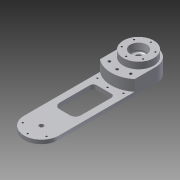
# Autodesk Inventor part: JointC2_2nd
Saved by Autodesk Inventor 2013 (Build 170138000, 138)
## iProperties
Created: 2013-02-07
Part Number: JointC2_2nd
Document SubType Name: Modeling
Designer: JohnHenry
Density: 0.899 g/cm^3
Material: ポリプロピレン
Mass: 21.971 g
Surface Area: 103.887 cm^2
Volume: 24.4394 cm^3
Author: JohnHenry
Autodesk Inventor part; units mm, degrees
ref_plane "YZ Plane" through (0, 0, 0) normal (1, 0, 0) x (0, 1, 0)
ref_plane "XZ Plane" through (0, 0, 0) normal (0, 1, 0) x (-1, 0, 0)
ref_plane "XY Plane" through (0, 0, 0) normal (0, 0, 1) x (1, 0, 0)
sketch "スケッチ1" plane through (0, 0, 0) normal (0, 0, 1) x (1, 0, 0)
  line L0 (-15.75, -60) -> (15.75, -60)
  line L1 (15.75, -60) -> (15.75, 60)
  line L2 (15.75, 60) -> (-15.75, 60)
  line L3 (-15.75, 60) -> (-15.75, -60)
  point P0 (0, 0)
  dimension "d0" = 31.5
  dimension "d1" = 15.75
  dimension "d2" = 120
  dimension "d3" = 60
  constraints: 8 end point, 2 parallel, 1 horizontal, 1 perpendicular
  measures "d0" distance of L1.end L2.end
  measures "d1" distance from line of L1 point (0, 0)
  measures "d2" distance of L2.end L0.start
  measures "d3" distance from line of L0 point (0, 0)
extrude "押し出し1" add sketch "スケッチ1" along normal blind 5
fillet "フィレット1" radius 15.75 4 edges at (-15.75, 60, 2.5) (15.75, 60, 2.5) (15.75, -60, 2.5) (-15.75, -60, 2.5)
sketch "スケッチ2" plane through (0, 0, 5) normal (0, 0, 1) x (1, 0, 0)
  arc A0 (15.75, 44.25) -> (-15.75, 44.25) centre (0, 44.25) ccw projected
  circle A1 centre (0, 44.25) radius 11.25
  point P0 (0, 0)
  point P1 (0, 55.5)
  point P2 (9.7428, 49.875)
  point P3 (9.7428, 38.625)
  point P4 (0, 33)
  point P5 (-9.7428, 38.625)
  point P6 (-9.7428, 49.875)
  dimension "d7" = 22.5
  dimension "d10" = 360
  constraints: 1 coincident, 1 vertical alignment, 9 other
hole "Hole1" at (0, 55.5, 5) at (9.7428, 49.875, 5) at (9.7428, 38.625, 5) at (0, 33, 5) at (-9.7428, 38.625, 5) at (-9.7428, 49.875, 5) direction (0, 0, -1) diameter 1.567 depth 8 tip angle 118 thread size "M2x0.4" class "6H" standard "ISO Metric profile"
sketch "スケッチ3" plane through (0, 0, 5) normal (0, 0, 1) x (1, 0, 0)
  arc A0 (15.75, 44.25) -> (-15.75, 44.25) centre (0, 44.25) ccw projected
  point P0 (0, 0)
  constraints: 1 coincident
hole "Hole2" at (0, 44.25, 5) direction (0, 0, -1) diameter 13 end through all
chamfer "面取り1" distance 1 distance2 5 1 edges at (0, 50.75, 5) measured on face at (0, -18.7612, 5)
sketch "スケッチ5" plane through (0, 0, 0) normal (0, 0, -1) x (-1, 0, 0)
  circle A0 centre (9.7428, 49.875) radius 0.7835 projected
  circle A1 centre (9.7428, 38.625) radius 0.7835 projected
  circle A2 centre (0, 33) radius 0.7835 projected
  circle A3 centre (-9.7428, 38.625) radius 0.7835 projected
  circle A4 centre (-9.7428, 49.875) radius 0.7835 projected
  circle A5 centre (0, 55.5) radius 0.7835 projected
  arc A6 (-15.75, -44.25) -> (15.75, -44.25) centre (0, -44.25) ccw projected
  line L0 (15.75, 44.25) -> (15.75, -44.25) projected
  arc A7 (15.75, 44.25) -> (-15.75, 44.25) centre (0, 44.25) ccw projected
  line L1 (-15.75, -44.25) -> (-15.75, 44.25) projected
  circle A8 centre (0, 44.25) radius 3
  point P0 (0, 0)
  dimension "d31" = 6
  constraints: 1 centre point, 1 coincident
  measures "d31" diameter of A8
extrude "押し出し3" add sketch "スケッチ5" along normal blind 15
sketch "スケッチ6" plane through (0, 44.25, 0) normal (0, 0, 1) x (1, 0, 0)
  circle A0 centre (0, 0) radius 3 projected
  circle A1 centre (0, 0) radius 6.5 projected
  point P0 (0, -44.25)
extrude "押し出し4" cut sketch "スケッチ6" against normal blind 1
sketch "スケッチ7" plane through (0, 44.25, -1) normal (0, 0, 1) x (1, 0, 0)
  circle A0 centre (0, 0) radius 6.5 projected
  circle A1 centre (0, 0) radius 4.5
  point P0 (0, -44.25)
  dimension "d36" = 9
  constraints: 1 centre point, 1 coincident
  measures "d36" diameter of A1
extrude "押し出し5" cut sketch "スケッチ7" against normal blind 1
fillet "フィレット2" radius 1 2 edges at (-6.5, 44.25, -2) (-4.5, 44.25, -2)
sketch "スケッチ9" plane through (0, 0, 5) normal (0, 0, 1) x (1, 0, 0)
  arc A0 (-15.75, -44.25) -> (15.75, -44.25) centre (0, -44.25) ccw projected
  line L0 (15.75, 44.25) -> (15.75, -44.25) projected
  arc A1 (15.75, 44.25) -> (-15.75, 44.25) centre (0, 44.25) ccw projected
  line L1 (-15.75, -44.25) -> (-15.75, 44.25) projected
  circle A2 centre (0, 44.25) radius 7.5 projected
  circle A3 centre (0, 44.25) radius 13.9
  point P0 (0, 0)
  dimension "d46" = 27.8
  constraints: 1 centre point, 1 coincident
  measures "d46" diameter of A3
extrude "押し出し7" cut sketch "スケッチ9" against normal blind 6 contours L1 A1 L0 A0
sketch "スケッチ10" plane through (0, 0, -1) normal (0, 0, 1) x (1, 0, 0)
  line L0 (15.75, 44.25) -> (15.75, -44.25) projected
  arc A0 (15.75, 44.25) -> (-15.75, 44.25) centre (0, 44.25) ccw projected
  line L1 (-15.75, -44.25) -> (-15.75, 44.25) projected
  arc A1 (-15.75, -44.25) -> (15.75, -44.25) centre (0, -44.25) ccw projected
  arc A2 (15.75, 24.8351) -> (-15.75, 24.8351) centre (0, 44.25) ccw
  arc A3 (-15.75, 24.8351) -> (15.75, 24.8351) centre (0, 44.25) ccw
  point P0 (0, 0)
  dimension "d49" = 50
  constraints: 4 point on circle, 2 centre point, 2 point on line, 1 coincident
  measures "d49" diameter of A2
extrude "押し出し8" cut sketch "スケッチ10" against normal blind 10 contours L0 A1 L1 A3
sketch "スケッチ11" plane through (0, 0, -11) normal (0, 0, 1) x (1, 0, 0)
  arc A0 (-15.75, -44.25) -> (15.75, -44.25) centre (0, -44.25) ccw projected
  point P0 (0, 0)
  constraints: 1 coincident
hole "Hole3" at (0, -44.25, -11) direction (0, 0, -1) diameter 4 end through all
sketch "スケッチ12" plane through (0, 0, -1) normal (0, 0, 1) x (1, 0, 0)
  line L0 (-15.75, 24.8351) -> (-15.75, 44.25) projected
  circle A0 centre (0, 44.25) radius 13.9 projected
  circle A1 centre (0, 44.25) radius 19.5
  line L1 (0, 44.25) -> (0, 63.75)
  line L2 (0, 44.25) -> (-9.75, 27.3625)
  line L3 (0, 44.25) -> (9.75, 27.3625)
  line L4 (15.75, 44.25) -> (15.75, 24.8351) projected
  arc A2 (15.75, 44.25) -> (-15.75, 44.25) centre (0, 44.25) ccw projected
  line L5 (0, 44.25) -> (0, 24.75)
  point P0 (0, 0)
  dimension "d59" = 39
  dimension "d60" = 150
  dimension "d61" = 150
  constraints: 8 end point, 4 coincident, 4 point on circle, 2 parallel, 1 centre point
  measures "d59" diameter of A1
  measures "d60" angle of L2 L1
  measures "d61" angle of L3 L1
hole "Hole4" at (-9.75, 27.3625, -1) at (9.75, 27.3625, -1) at (0, 24.75, -1) direction (0, 0, -1) diameter 2.459 end through all thread size "M3x0.5" class "6H" standard "ISO Metric profile"
sketch "スケッチ14" plane through (0, 0, -11) normal (0, 0, 1) x (1, 0, 0)
  circle A0 centre (0, -44.25) radius 2 projected
  arc A1 (-15.75, 24.8351) -> (15.75, 24.8351) centre (0, 44.25) ccw projected
  arc A2 (-15.75, -44.25) -> (15.75, -44.25) centre (0, -44.25) ccw projected
  line L0 (-9.85, 12.8) -> (9.85, 12.8)
  line L1 (9.85, 12.8) -> (9.85, -23.1)
  line L2 (9.85, -23.1) -> (-9.85, -23.1)
  line L3 (-9.85, -23.1) -> (-9.85, 12.8)
  line L4 (0, 19.25) -> (0, -60)
  point P0 (0, 0)
  dimension "d77" = 19.7
  dimension "d78" = 19.7
  dimension "d79" = 35.9
  dimension "d80" = 21.15
  constraints: 10 end point, 2 parallel, 2 point on circle, 1 horizontal, 1 perpendicular
  measures "d77" distance of L0.start L0.end
  measures "d78" diameter of L1 L4
  measures "d79" distance between parallel lines of L2 L0
  measures "d80" distance from line of A0.centre L2
extrude "押し出し9" cut sketch "スケッチ14" against normal through all contours L0 L4 L2 L3 | L0 L1 L2 L4
fillet "フィレット3" radius 5.05 2 edges at (-9.85, -23.1, -13) (9.85, -23.1, -13)
fillet "フィレット4" radius 3.05 2 edges at (-9.85, 12.8, -13) (9.85, 12.8, -13)
sketch "スケッチ15" plane through (0, 0, -11) normal (0, 0, 1) x (1, 0, 0)
  line L0 (-6.8, 12.8) -> (6.8, 12.8) projected
  circle A0 centre (0, -44.25) radius 2 projected
  line L1 (15.75, 24.8351) -> (15.75, -44.25) projected
  circle A1 centre (0, 44.25) radius 31.45
  line L2 (0, 19.25) -> (0, 12.8)
  circle A2 centre (0, 44.25) radius 28.225
  line L3 (0, 44.25) -> (0, 12.8)
  line L4 (0, 44.25) -> (-11.9284, 18.6695)
  line L5 (0, 44.25) -> (11.9284, 18.6695)
  circle A3 centre (0, -44.25) radius 12.5
  line L6 (0, -44.25) -> (0, -56.75)
  line L7 (0, -44.25) -> (10.8253, -50.5)
  line L8 (0, -44.25) -> (-10.8253, -50.5)
  point P0 (0, 0)
  point P1 (0, 16.025)
  point P2 (10.8253, -50.5)
  dimension "d86" = 25
  dimension "d87" = 25
  dimension "d88" = 25
  dimension "d93" = 120
  dimension "d94" = 60
  dimension "d95" = 180
  dimension "d96" = 0
  dimension "d97" = 0
  constraints: 14 end point, 5 coincident, 5 point on circle, 4 point on line, 2 centre point, 1 collinear, 1 midpoint, 1 vertical alignment, 2 other
  measures "d86" angle of L4 L3
  measures "d87" angle of L3 L5
  measures "d88" diameter of A3
  measures "d93" angle of L8 L7
  measures "d94" angle of L8 L6
  measures "d95" angle of L1 L6
  measures "d96" distance of A3.centre A0.centre
  measures "d97" distance of A3.centre A0.centre
hole "Hole6" at (0, -44.25, -11) at (-11.9284, 18.6695, -11) at (0, 16.025, -11) at (11.9284, 18.6695, -11) at (10.8253, -50.5, -11) at (0, -56.75, -11) at (-10.8253, -50.5, -11) direction (0, 0, -1) diameter 1.567 depth 8 tip angle 118 thread size "M2x0.4" class "6H" standard "ISO Metric profile"
chamfer "面取り2" distance 0.5 angle 45 4 edges at (-15.75, 0, -15) (0, -60, -15) (15.75, 0, -15) (0, 60, -15)
equation "\"d1\" = 0.5 * d0"
equation "\"d3\" = 0.5 * d2"
equation "\"d60\" = d61"
equation "\"d78\" = d77"
equation "\"d94\" = 0.5 * d93"
